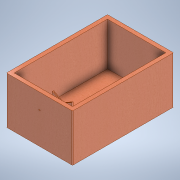
# Autodesk Inventor part: BoxDark
Saved by Autodesk Inventor 2022.2 (Build 262287010, 287A)
## iProperties
Created: 2022-03-17
Part Number: BoxDark
Material: Genérico
Document SubType Name: Modeling
Designer: mabel
Density: 1 g/cm^3
Appearance: Nogal - Natural pulido
Author: mabel
Autodesk Inventor part; units mm, degrees
ref_plane "YZ Plane" through (0, 0, 0) normal (1, 0, 0) x (0, 1, 0)
ref_plane "XZ Plane" through (0, 0, 0) normal (0, 1, 0) x (-1, 0, 0)
ref_plane "XY Plane" through (0, 0, 0) normal (0, 0, 1) x (1, 0, 0)
sketch "Boceto1" plane through (0, 0, 0) normal (0, 1, 0) x (-1, 0, 0)
  line L0 (-85, -130) -> (85, -130)
  line L1 (85, -130) -> (85, 130)
  line L2 (85, 130) -> (-85, 130)
  line L3 (-85, 130) -> (-85, -130)
  line L4 (-85, -130) -> (85, 130) construction
  line L5 (85, -130) -> (-85, 130) construction
  line L6 (75, 120) -> (75, -120)
  line L7 (75, -120) -> (-75, -120)
  line L8 (-75, -120) -> (-75, 120)
  line L9 (-75, 120) -> (75, 120)
  point P0 (0, 0)
  point P1 (0, -120)
  point P2 (0, 120)
  point P3 (0, 0)
  dimension "d0" = 170
  dimension "d1" = 260
  dimension "d10" = 10
  constraints: 20 end point, 5 midpoint, 4 parallel, 2 perpendicular, 1 horizontal, 3 other
  measures "d0" distance of L2.end L1.end
  measures "d1" distance of L1.end L0.end
  measures "d10" distance between parallel lines of L1 L6
extrude "Extrusión1" add sketch "Boceto1" along normal blind 121
extrude "Extrusión3" add sketch "Boceto1" along normal blind 10 contours L6 L7 L8 L9
sketch "Boceto4" plane through (0, 10, 0) normal (0, 1, 0) x (1, 0, 0)
  circle A0 centre (0, 4.19) radius 3.75
  line L0 (85, 130) -> (-85, 130) projected
  circle A1 centre (0, 4.19) radius 3.35
  circle A2 centre (0, 4.19) radius 1.5
  line L1 (-85, -130) -> (85, -130) projected
  line L2 (75, -120) -> (-75, -120) construction
  line L3 (0, -120) -> (0, -70) construction
  point P0 (0, 0)
  dimension "d15" = 7.5
  dimension "d17" = 0.4
  dimension "d20" = 3
  dimension "d23" = 134.19
  dimension "d36" = 50
  constraints: 3 centre point, 2 end point, 1 coincident, 1 midpoint, 1 vertical
  measures "d15" diameter of A0
  measures "d17" radial gap between concentric circles of A0 A1
  measures "d20" diameter of A2
  measures "d23" distance from line of A0.centre L1
  measures "d36" distance of L3.start L3.end
extrude "Extrusión4" add sketch "Boceto4" along normal blind 21 contours A0
extrude "Extrusión5" cut sketch "Boceto4" against normal blind 10 contours A2
sketch "Boceto7" plane through (0, 10, 0) normal (0, 1, 0) x (1, 0, 0)
  circle A0 centre (0, 4.19) radius 1.5 construction
  line L0 (0, 4.19) -> (-17.5, 4.19) construction
  circle A1 centre (0, 4.19) radius 1.5 construction
  line L1 (0, 4.19) -> (0, -27.68) construction
  line L2 (75, -120) -> (-75, -120) construction
  line L3 (0, -120) -> (0, -70) construction
  line L4 (0, -70) -> (-19.0745, -70) construction
  line L5 (25, -68) -> (-25, -68)
  line L6 (-25, -68) -> (-25, -72)
  line L7 (-25, -72) -> (25, -72)
  line L8 (25, -72) -> (25, -68)
  line L9 (25, -68) -> (-25, -72) construction
  line L10 (-25, -68) -> (25, -72) construction
  line L11 (-23.5, -70.5) -> (-23.5, -69.5)
  line L12 (-23.5, -69.5) -> (23.5, -69.5)
  line L13 (23.5, -69.5) -> (23.5, -70.5)
  line L14 (23.5, -70.5) -> (-23.5, -70.5)
  line L15 (-4.25, -22.43) -> (-17.75, -22.43)
  line L16 (-17.75, -22.43) -> (-17.75, -27.93)
  line L17 (-17.75, -27.93) -> (-4.25, -27.93)
  line L18 (-4.25, -27.93) -> (-4.25, -22.43)
  line L19 (17.75, -22.43) -> (4.25, -22.43)
  line L20 (4.25, -22.43) -> (4.25, -27.93)
  line L21 (4.25, -27.93) -> (17.75, -27.93)
  line L22 (17.75, -27.93) -> (17.75, -22.43)
  line L23 (-4.25, 36.31) -> (-17.75, 36.31)
  line L24 (-17.75, 36.31) -> (-17.75, 30.81)
  line L25 (-17.75, 30.81) -> (-4.25, 30.81)
  line L26 (-4.25, 30.81) -> (-4.25, 36.31)
  line L27 (18.25, 36.31) -> (4.75, 36.31)
  line L28 (4.75, 36.31) -> (4.75, 30.81)
  line L29 (4.75, 30.81) -> (18.25, 30.81)
  line L30 (18.25, 30.81) -> (18.25, 36.31)
  point P0 (0, 0)
  dimension "d43" = 31.87
  dimension "d44" = 50
  dimension "d45" = 50
  dimension "d46" = 4
  dimension "d47" = 1.5
  dimension "d100" = 13.5
  dimension "d101" = 5.5
  dimension "d102" = 13.5
  dimension "d103" = 5.5
  dimension "d104" = 13.5
  dimension "d105" = 5.5
  dimension "d106" = 13.5
  dimension "d107" = 5.5
  constraints: 60 end point, 12 parallel, 7 perpendicular, 6 horizontal, 3 midpoint, 2 vertical, 3 other
  measures "d43" distance of L1.start L1.end
  measures "d44" distance of L3.start L3.end
  measures "d45" distance of L7.end L6.end
  measures "d46" distance of L6.end L5.end
  measures "d47" distance between parallel lines of L6 L11
  measures "d100" distance of L17.end L16.end
  measures "d101" distance of L16.end L15.end
  measures "d102" distance of L21.end L20.end
  measures "d103" distance of L20.end L19.end
  measures "d104" distance of L25.end L24.end
  measures "d105" distance of L24.end L23.end
  measures "d106" distance of L29.end L28.end
  measures "d107" distance of L28.end L27.end
sketch "Boceto8" plane through (75, 121, 120) normal (0, 0, -1) x (-1, 0, 0)
  line L0 (0, -111) -> (150, -111) construction
  line L1 (75, -111) -> (75, -11) construction
  circle A0 centre (75, -40) radius 5
  circle A1 centre (75, -40) radius 1.5
  point P0 (75, -121)
  dimension "d37" = 100
  dimension "d38" = 10
  dimension "d75" = 3
  constraints: 2 centre point, 2 end point, 1 coincident, 1 midpoint, 1 vertical
  measures "d37" distance of L1.start L1.end
  measures "d38" diameter of A0
  measures "d75" diameter of A1
extrude "Extrusión9" add sketch "Boceto7" along normal blind 71 contours L8 L7 L6 L5
sketch "Boceto9" plane through (-25, 10, 72) normal (0, 0, 1) x (1, 0, 0)
  line L0 (0, 71) -> (25, 56.5662)
  line L1 (0, 71) -> (57.416, 71) construction
  line L2 (50, 71) -> (25, 56.5662)
  line L3 (50, 71) -> (104.7106, 71) construction
  arc A0 (48.8838, 70.3556) -> (1.1162, 70.3556) centre (25, 56.5662) ccw
  line L4 (0, 71) -> (1.5, 71)
  line L5 (0, 71) -> (50, 71) projected
  line L6 (50, 71) -> (48.5, 71)
  point P0 (25, -10)
  constraints: 12 end point, 4 point on circle, 3 point on line, 2 horizontal, 1 centre point, 1 coincident, 1 collinear
extrude "Extrusión11" add sketch "Boceto9" against normal blind 4 contours A0 L5 L2 L0 | A0 L5
extrude "Extrusión12" cut sketch "Boceto9" against normal blind 4 contours A0 L5 L2 L0 | A0 L5
extrude "Extrusión13" cut sketch "Boceto9" against normal blind 4 contours L4 A0 L0
extrude "Extrusión14" cut sketch "Boceto9" against normal blind 4 contours L5 L2 A0
extrude "Extrusión15" [suppressed]
extrude "Extrusión16" [suppressed]
fillet "Empalme1" radius 2 4 edges at (85, 60.5, 130) (-85, 60.5, 130) (85, 60.5, -130) (-85, 60.5, -130)
extrude "Extrusión17" cut sketch "Boceto8" against normal through all contours A1
extrude "Extrusión20" cut sketch "Boceto7" against normal blind 5 contours L18 L17 L16 L15 | L22 L21 L20 L19 | L26 L25 L24 L23 | L30 L29 L28 L27
